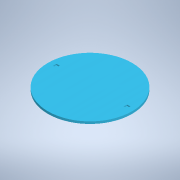
# Autodesk Inventor part: pat
Saved by Autodesk Inventor 2022 (Build 260153000, 153)
## iProperties
Created: 2022-02-27
Part Number: pat
Material: PET Plastic
Document SubType Name: Modeling
Designer: Oana
Density: 1.541 g/cm^3
Appearance: Turquoise
Author: Oana
Autodesk Inventor part; units mm, degrees
ref_plane "YZ Plane" through (0, 0, 0) normal (1, 0, 0) x (0, 1, 0)
ref_plane "XZ Plane" through (0, 0, 0) normal (0, 1, 0) x (-1, 0, 0)
ref_plane "XY Plane" through (0, 0, 0) normal (0, 0, 1) x (1, 0, 0)
sketch "Sketch1" plane through (0, 0, 0) normal (0, 1, 0) x (-1, 0, 0)
  circle A0 centre (0, 0) radius 75
  dimension "d0" = 150
  constraints: 1 centre point, 1 coincident
  measures "d0" diameter of A0
extrude "Extrusion1" add sketch "Sketch1" along normal blind 4
sketch "Sketch2" plane through (0, 0, 0) normal (0, -1, 0) x (1, 0, 0)
  point P0 (0, 0)
sketch "Sketch4" plane through (0, 0, 0) normal (0, -1, 0) x (1, 0, 0)
  circle A0 centre (0, 0) radius 5.5
  dimension "d7" = 11
  constraints: 1 centre point, 1 coincident
  measures "d7" diameter of A0
extrude "Extrusion3" add sketch "Sketch4" along normal blind 5
sketch "Sketch5" plane through (0, 0, 0) normal (0, -1, 0) x (1, 0, 0)
  point P0 (0, 0)
sketch "Sketch8" plane through (0, -5, 0) normal (0, -1, 0) x (1, 0, 0)
  line L0 (3.9692, 4.8706) -> (31.1403, 4.8706)
  line L1 (31.1403, 4.8706) -> (31.1403, -5.1294)
  line L2 (31.1403, -5.1294) -> (3.9692, -5.1294)
  line L3 (3.9692, -5.1294) -> (3.9692, 4.8706)
  point P0 (0, 0)
  dimension "d15" = 10
  constraints: 8 end point, 2 parallel, 1 horizontal, 1 perpendicular
  measures "d15" distance of L2.end L0.start
extrude "Extrusion5" cut sketch "Sketch8" against normal blind 1
sketch "Sketch9" plane through (0, 0, 0) normal (0, -1, 0) x (1, 0, 0)
  circle A0 centre (-24.5, 0) radius 1.5 construction
  circle A1 centre (0, 28.5) radius 1.5 construction
  circle A2 centre (0, -28.5) radius 1.5 construction
  circle A3 centre (0, -28.5) radius 2
  circle A4 centre (-24.5, 0) radius 2
  circle A5 centre (0, 28.5) radius 2
  point P0 (0, 0)
  dimension "d28" = 4
  dimension "d29" = 4
  dimension "d30" = 4
  constraints: 3 centre point, 3 coincident
  measures "d28" diameter of A3
  measures "d29" diameter of A4
  measures "d30" diameter of A5
extrude "Extrusion6" cut sketch "Sketch9" against normal blind 2
sketch "Sketch10" plane through (0, 4, 0) normal (0, 1, 0) x (1, 0, 0)
  line L0 (0, 0) -> (-8.5469, 0)
  line L1 (-66, 0) -> (-60, 0)
  line L2 (-60, 0) -> (-60, 6)
  line L3 (-60, 6) -> (-66, 6)
  line L4 (-66, 6) -> (-66, 0)
  line L5 (60, 6) -> (66, 6)
  line L6 (66, 6) -> (66, 0)
  line L7 (66, 0) -> (60, 0)
  line L8 (60, 0) -> (60, 6)
  line L9 (-60, 3) -> (0, 3)
  line L10 (0, 0) -> (0, 26.4138)
  line L11 (60, 3) -> (0, 3)
  line L12 (0, 0) -> (22.9317, 0)
  dimension "d22" = 6
  dimension "d23" = 6
  dimension "d24" = 60
  constraints: 26 end point, 4 horizontal, 4 parallel, 4 perpendicular, 3 equal length, 2 midpoint, 2 vertical, 1 point on line
  measures "d22" distance of L2.end L3.end
  measures "d23" distance of L1.end L2.end
  measures "d24" distance of L9.start L9.end
extrude "Extrusion7" cut sketch "Sketch10" against normal blind 2
equation "\"d0\" = diamteru"
equation "\"d1\" = grosime"
equation "\"diamteru\" = 150"
equation "\"grosime\" = 4"
body "Solid1"
